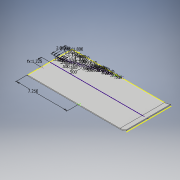
# Autodesk Inventor part: Part2
Saved by Autodesk Inventor 2018 (Build 220112000, 112)
## iProperties
Created: 2018-03-02
Part Number: Part2
Material: Generic
Document SubType Name: Modeling
Designer: 232963
Density: 1 g/cm^3
Appearance: Default
Author: 232963
Autodesk Inventor part; units mm, degrees
ref_plane "YZ Plane" through (0, 0, 0) normal (1, 0, 0) x (0, 1, 0)
ref_plane "XZ Plane" through (0, 0, 0) normal (0, 1, 0) x (-1, 0, 0)
ref_plane "XY Plane" through (0, 0, 0) normal (0, 0, 1) x (1, 0, 0)
sketch "Sketch1" plane through (0, 0, 0) normal (0, 0, 1) x (1, 0, 0)
  line L0 (-24.821, 0) -> (308.554, 0)
  line L1 (330.779, 6.35) -> (330.779, 9.144)
  line L2 (-24.821, 2.794) -> (-24.821, 0)
  arc A0 (308.554, 2.794) -> (330.779, 9.144) centre (308.4605, 45.1902) ccw
  arc A1 (308.554, 0) -> (330.779, 6.35) centre (308.4605, 42.3962) ccw
  line L3 (-24.821, 2.794) -> (308.554, 2.794)
  point P0 (0, 0)
  constraints: 8 end point, 4 point on circle, 2 centre point, 1 horizontal, 1 parallel, 1 perpendicular, 1 other
extrude "Extrusion1" add sketch "Sketch1" along normal blind 160.3375
sketch "Sketch2" plane through (-24.821, 2.794, 0) normal (0, 1, 0) x (1, 0, 0)
  line L0 (355.6, 0) -> (355.6, -160.3375) projected
  line L1 (0, 0) -> (0, -160.3375) projected
  line L2 (0, -80.1688) -> (355.6, -80.1688)
  line L3 (333.375, 0) -> (0, 0) projected
  line L4 (0, 0) -> (333.375, 0) projected
  point P0 (24.821, 0)
  point P1 (0, -111.2838)
  point P2 (184.15, -160.3375)
  point P3 (0, -52.4002)
  point P4 (6.35, -50.8)
  point P5 (12.7, -49.6824)
  point P6 (19.05, -47.244)
  point P7 (25.4, -45.72)
  point P8 (63.5, -33.02)
  point P9 (31.75, -44.45)
  point P10 (38.1, -41.91)
  point P11 (50.8, -36.83)
  point P12 (76.2, -27.94)
  point P13 (88.9, -24.13)
  point P14 (101.6, -19.05)
  point P15 (114.3, -13.97)
  point P16 (127, -10.16)
  point P17 (139.7, -7.62)
  point P18 (152.4, -3.81)
  point P19 (165.1, -2.54)
  point P20 (177.8, 0)
  point P21 (44.45, -39.37)
  point P22 (69.85, -30.48)
  point P23 (82.55, -25.4)
  point P24 (95.25, -21.59)
  point P25 (107.95, -16.51)
  point P26 (120.65, -12.7)
  point P27 (133.35, -8.89)
  point P28 (146.05, -5.08)
  point P29 (159.4552, -4.424)
  point P30 (171.2115, -1.9186)
  point P31 (57.15, -35.56)
  dimension "d8" = 31.115
  dimension "d9" = 184.15
  dimension "d12" = 52.4002
  dimension "d13" = 50.8
  dimension "d14" = 49.6824
  dimension "d15" = 47.244
  dimension "d16" = 6.35
  dimension "d17" = 6.35
  dimension "d18" = 6.35
  dimension "d19" = 6.35
  dimension "d20" = 45.72
  dimension "d29" = 44.45
  dimension "d30" = 6.35
  dimension "d31" = 41.91
  dimension "d32" = 36.83
  dimension "d33" = 12.7
  dimension "d34" = 6.35
  dimension "d35" = 33.02
  dimension "d36" = 12.7
  dimension "d37" = 27.94
  dimension "d38" = 12.7
  dimension "d39" = 24.13
  dimension "d40" = 19.05
  dimension "d41" = 12.7
  dimension "d42" = 12.7
  dimension "d43" = 13.97
  dimension "d44" = 12.7
  dimension "d45" = 10.16
  dimension "d46" = 12.7
  dimension "d47" = 7.62
  dimension "d48" = 12.7
  dimension "d49" = 3.81
  dimension "d50" = 12.7
  dimension "d51" = 2.54
  dimension "d52" = 12.7
  dimension "d53" = 12.7
  dimension "d54" = 39.37
  dimension "d55" = 6.35
  dimension "d56" = 35.56
  dimension "d57" = 30.48
  dimension "d58" = 6.35
  dimension "d59" = 6.35
  dimension "d60" = 25.4
  dimension "d61" = 6.35
  dimension "d62" = 21.59
  dimension "d63" = 6.35
  dimension "d64" = 16.51
  dimension "d65" = 12.7
  dimension "d66" = 6.35
  dimension "d67" = 6.35
  dimension "d68" = 8.89
  dimension "d69" = 6.35
  dimension "d70" = 5.08
  dimension "d71" = 6.35
  constraints: 3 point on line, 2 end point, 2 midpoint
  measures "d8" distance of point (0, -111.284) L2.start
  measures "d9" distance of L1.end point (184.15, -160.338)
  measures "d12" distance from line of L3 point (0, -52.4)
  measures "d13" distance from line of L3 point (6.35, -50.8)
  measures "d14" distance from line of L3 point (12.7, -49.682)
  measures "d15" distance from line of L3 point (19.05, -47.244)
  measures "d16" horizontal distance of point (6.35, -50.8) point (0, -52.4)
  measures "d17" horizontal distance of point (12.7, -49.682) point (6.35, -50.8)
  measures "d18" horizontal distance of point (12.7, -49.682) point (19.05, -47.244)
  measures "d19" horizontal distance of point (25.4, -45.72) point (19.05, -47.244)
  measures "d20" distance from line of L3 point (25.4, -45.72)
  measures "d29" distance from line of L3 point (31.75, -44.45)
  measures "d30" horizontal distance of point (31.75, -44.45) point (25.4, -45.72)
  measures "d31" distance from line of L3 point (38.1, -41.91)
  measures "d32" distance from line of L3 point (50.8, -36.83)
  measures "d33" horizontal distance of point (38.1, -41.91) point (50.8, -36.83)
  measures "d34" horizontal distance of point (38.1, -41.91) point (31.75, -44.45)
  measures "d35" distance from line of L3 point (63.5, -33.02)
  measures "d36" horizontal distance of point (50.8, -36.83) point (63.5, -33.02)
  measures "d37" distance from line of L3 point (76.2, -27.94)
  measures "d38" horizontal distance of point (63.5, -33.02) point (76.2, -27.94)
  measures "d39" distance from line of L3 point (88.9, -24.13)
  measures "d40" distance from line of L3 point (101.6, -19.05)
  measures "d41" horizontal distance of point (88.9, -24.13) point (76.2, -27.94)
  measures "d42" horizontal distance of point (88.9, -24.13) point (101.6, -19.05)
  measures "d43" distance from line of L3 point (114.3, -13.97)
  measures "d44" horizontal distance of point (101.6, -19.05) point (114.3, -13.97)
  measures "d45" distance from line of L3 point (127, -10.16)
  measures "d46" horizontal distance of point (114.3, -13.97) point (127, -10.16)
  measures "d47" distance from line of L3 point (139.7, -7.62)
  measures "d48" horizontal distance of point (127, -10.16) point (139.7, -7.62)
  measures "d49" distance from line of L3 point (152.4, -3.81)
  measures "d50" horizontal distance of point (139.7, -7.62) point (152.4, -3.81)
  measures "d51" distance from line of L3 point (165.1, -2.54)
  measures "d52" horizontal distance of point (152.4, -3.81) point (165.1, -2.54)
  measures "d53" horizontal distance of point (165.1, -2.54) point (177.8, 0)
  measures "d54" distance from line of point (44.45, -39.37) L4
  measures "d55" horizontal distance of point (38.1, -41.91) point (44.45, -39.37)
  measures "d56" distance from line of L3 point (57.15, -35.56)
  measures "d57" distance from line of L3 point (69.85, -30.48)
  measures "d58" horizontal distance of point (76.2, -27.94) point (69.85, -30.48)
  measures "d59" horizontal distance of point (50.8, -36.83) point (57.15, -35.56)
  measures "d60" distance from line of L3 point (82.55, -25.4)
  measures "d61" horizontal distance of point (88.9, -24.13) point (82.55, -25.4)
  measures "d62" distance from line of L3 point (95.25, -21.59)
  measures "d63" horizontal distance of point (88.9, -24.13) point (95.25, -21.59)
  measures "d64" distance from line of L3 point (107.95, -16.51)
  measures "d65" distance from line of L3 point (120.65, -12.7)
  measures "d66" horizontal distance of point (114.3, -13.97) point (120.65, -12.7)
  measures "d67" horizontal distance of point (101.6, -19.05) point (107.95, -16.51)
  measures "d68" distance from line of L3 point (133.35, -8.89)
  measures "d69" horizontal distance of point (127, -10.16) point (133.35, -8.89)
  measures "d70" distance from line of L3 point (146.05, -5.08)
  measures "d71" horizontal distance of point (139.7, -7.62) point (146.05, -5.08)
equation "\"d8\" = d7"
equation "\"d7\" = 31.115"
body "Solid1"
